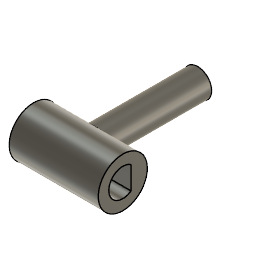
rotary (Autodesk Fusion 360 design; units mm, degrees)
part number: 2026-05-17-21-40-16-514
Autodesk Fusion 360 part; units mm, degrees
sketch "Sketch1" plane through (0, 0, 0) normal (0, 0, 1) x (1, 0, 0)
  circle A0 centre (0, 0) radius 7
  circle A1 centre (0, 0) radius 4
  line L0 (-3.2536, 2.3268) -> (3.2464, 2.3369)
  dimension "d1" = 14
  dimension "d2" = 8
  dimension "d3" = 6.5
  constraint coincident A0.centre A1.centre
  constraint coincident A1 L0.start
  constraint coincident A1 L0.end
  measures "d1" diameter of A0
  measures "d2" diameter of A1
  measures "d3" distance of L0.start L0.end
extrude "Extrude1" add sketch "Sketch1" along normal blind 25.4 contours A0 | A1 L0 picked at (-0.9258, 2.9951) makes body 1
sketch "Sketch2" plane through (-0.0036, 2.3318, 0) normal (0.00156, -0.999999, 0) x (0.999999, 0.00156, 0)
  line L0 (-3.25, 0) -> (3.25, 0)
  line L1 (3.25, 0) -> (3.25, 25.4)
  line L2 (3.25, 25.4) -> (-3.25, 25.4)
  line L3 (-3.25, 25.4) -> (-3.25, 0)
  circle A0 centre (0, 14) radius 4
  dimension "d6" = 8
  measures "d6" diameter of A0
extrude "Extrude2" add sketch "Sketch2" against normal blind 32 separate body contours L3 A0 | L1 L3 A0 | L1 A0 makes body 2
move_body "Move1" bodies 2 to x (1, 0, 0) y (0, 1, 0) z (0, 0, 1) at (0, 1, 0)
combine "Combine1" operation add target body 2 tool bodies 1
move_body "Move2" bodies 2 to x (0, 0, 1) y (0, 1, 0) z (-1, 0, 0) at (0, 0, 0)
move_body "Move3" bodies 2 to x (1, 0, 0) y (0, 1, 0) z (0, 0, 1) at (0, 0, 7)
